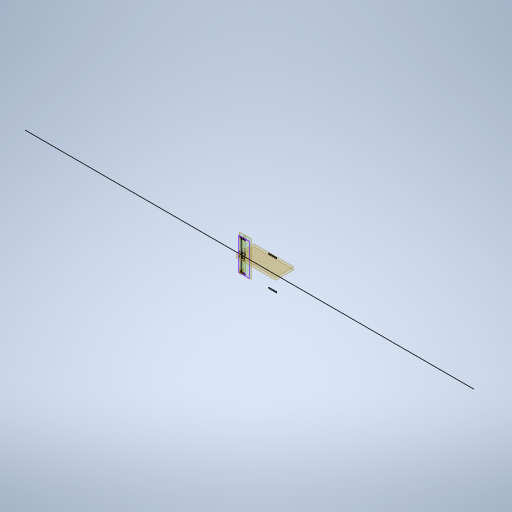
# Autodesk Inventor part: 4s
Saved by Autodesk Inventor 2024.2 (Build 282272000, 272)
## iProperties
Created: 2026-01-09
Part Number: 4s
Material: Типовые
Document SubType Name: Modeling
Designer: Service
Density: 1 g/cm^3
Appearance: По умолчанию
Author: Service
Autodesk Inventor part; units mm, degrees
ref_plane "YZ Plane" through (0, 0, 0) normal (1, 0, 0) x (0, 1, 0)
ref_plane "XZ Plane" through (0, 0, 0) normal (0, 1, 0) x (-1, 0, 0)
ref_plane "XY Plane" through (0, 0, 0) normal (0, 0, 1) x (1, 0, 0)
ref_plane "РабПлоскость1" through (0, 0, 0) normal (0, 0, 1) x (1, 0, 0)
sketch "Эскиз1" plane through (0, 0, 0) normal (0, 0, 1) x (1, 0, 0)
  line L0 (-20.21, 188.9707) -> (47.0583, 188.9707)
  line L1 (47.0583, 188.9707) -> (47.0583, -13.1291)
  line L2 (47.0583, -13.1291) -> (-20.21, -13.1291)
  line L3 (-20.21, -13.1291) -> (-20.21, 188.9707)
  line L4 (220, -6) -> (168.1947, -6)
  line L5 (168.1947, 0) -> (168.1947, -6)
  line L6 (168.1947, 0) -> (220, 0)
  line L7 (220, 0) -> (220, -6)
  line L8 (9.8053, -6) -> (-12, -6)
  line L9 (-12, -6) -> (-12, 0)
  line L10 (-12, 0) -> (9.8053, 0)
  line L11 (9.8053, 0) -> (9.8053, -6)
  line L12 (220, 180) -> (168.1947, 180)
  line L13 (168.1947, 186) -> (168.1947, 180)
  line L14 (168.1947, 186) -> (220, 186)
  line L15 (220, 186) -> (220, 180)
  line L16 (9.8053, 180) -> (-12, 180)
  line L17 (-12, 180) -> (-12, 186)
  line L18 (-12, 186) -> (9.8053, 186)
  line L19 (9.8053, 186) -> (9.8053, 180)
  line L20 (0, 180) -> (0, 0)
  line L21 (0, 0) -> (-6, 0)
  line L22 (-6, 0) -> (-6, 180)
  line L23 (-6, 180) -> (0, 180)
  circle A0 centre (-3, 175) radius 1.5
  circle A1 centre (-3, 5) radius 1.5
  line L24 (9.8053, -6) -> (24.8871, -6)
  line L25 (24.8871, -6) -> (24.8871, 0)
  line L26 (24.8871, 0) -> (9.8053, 0)
  line L27 (9.8053, 0) -> (9.8053, -6)
  line L28 (9.8053, 180) -> (24.8871, 180)
  line L29 (24.8871, 180) -> (24.8871, 188.9707)
  line L30 (24.8871, 188.9707) -> (9.8053, 188.9707)
  line L31 (9.8053, 188.9707) -> (9.8053, 180)
  circle A2 centre (6, 75) radius 1.5
  circle A3 centre (6, 105) radius 1.5
  line L32 (-1364.1034, 90) -> (1460.214, 90)
  line L33 (9.8053, 186) -> (24.8871, 186)
  dimension "d0" = 3
  dimension "d1" = 3
  dimension "d2" = 6
  dimension "d3" = 6
  dimension "d4" = 15
  dimension "d5" = 15
  constraints: 68 end point, 14 horizontal, 10 vertical, 6 parallel, 4 centre point, 4 perpendicular, 3 point on line, 25 other
  measures "d0" diameter of A3
  measures "d1" diameter of A2
  measures "d2" distance from line of L20 A2.centre
  measures "d3" distance from line of L20 A3.centre
  measures "d4" distance from line of L32 A2.centre
  measures "d5" distance from line of L32 A3.centre
ref_plane "РабПлоскость2" through (104, 75, -42) normal (0, 1, 0) x (-1, 0, 0)
sketch "Эскиз2" plane through (104, 75, -42) normal (0, 1, 0) x (-1, 0, 0)
  line L0 (104, 42) -> (104, 26.1085)
  line L1 (104, 26.1085) -> (90.5759, 39.2974)
  line L2 (90.5759, 39.2974) -> (104, 39.2974)
  constraints: 6 end point, 1 perpendicular, 1 point on line, 1 vertical
extrude "Выдавливание2" add sketch "Эскиз2" along normal mid plane 30
ref_plane "РабПлоскость3" through (104, 90, -42) normal (0, 1, 0) x (-1, 0, 0)
mirror "Зеркальное отражение1" about plane through (104, 90, -42) normal (0, 1, 0) of "Выдавливание2"
ref_plane "РабПлоскость7" through (0, 0, 0) normal (0, 0, 1) x (1, 0, 0)
sketch "Эскиз3" plane through (0, 0, 0) normal (0, 0, 1) x (1, 0, 0)
  line L0 (47.0583, 188.9707) -> (-20.21, 188.9707) projected
  line L1 (-20.21, 188.9707) -> (-20.21, -13.1291) projected
  line L2 (-20.21, -13.1291) -> (47.0583, -13.1291) projected
  line L3 (47.0583, -13.1291) -> (47.0583, 188.9707) projected
  circle A0 centre (6, 105) radius 1.5 projected
  circle A1 centre (6, 75) radius 1.5 projected
  line L4 (-12, 186) -> (24.8871, 186) projected
  line L5 (24.8871, 186) -> (24.8871, 180) projected
  line L6 (24.8871, 180) -> (0, 180) projected
  line L7 (0, 180) -> (0, 0) projected
  line L8 (0, 0) -> (24.8871, 0) projected
  line L9 (24.8871, 0) -> (24.8871, -6) projected
  line L10 (24.8871, -6) -> (-12, -6) projected
  line L11 (-12, -6) -> (-12, 0) projected
  line L12 (-12, 0) -> (-6, 0) projected
  line L13 (-6, 0) -> (-6, 180) projected
  line L14 (-6, 180) -> (-12, 180) projected
  line L15 (-12, 180) -> (-12, 186) projected
extrude "Выдавливание3" cut sketch "Эскиз3" against normal blind 13.891 contours A0 | A1
ref_plane "РабПлоскость4" through (0, 0, -10) normal (0, 0, -1) x (-1, 0, 0)
sketch "Эскиз4" plane through (0, 0, -10) normal (0, 0, -1) x (-1, 0, 0)
  line L0 (0, 60) -> (-13.4241, 60) projected
  line L1 (0, 120) -> (0, 60) projected
  line L2 (0, 120) -> (-13.4241, 120) projected
  circle A0 centre (-6, 105) radius 3.0499
  line L3 (-13.4241, 60) -> (-13.4241, 120) projected
  point P0 (0, 0)
  constraints: 1 centre point
extrude "Выдавливание4" cut sketch "Эскиз4" along normal blind 30 contours A0
mirror "Зеркальное отражение2" about plane through (104, 90, -42) normal (0, 1, 0) of "Выдавливание4"
ref_plane "РабПлоскость6" through (0, 0, 0) normal (-1, 0, 0) x (0, 0, 1)
sketch "Эскиз5" plane through (0, 0, 0) normal (-1, 0, 0) x (0, 0, 1)
  circle A0 centre (-10, 95) radius 1.3
  circle A1 centre (-10, 85) radius 1.3
  line L0 (-19.0698, 90) -> (3.1783, 90) projected
  line L1 (-3, -13.1291) -> (-3, 188.9707) projected
  point P0 (0, 0)
  dimension "d16" = 2.6
  dimension "d17" = 5
  dimension "d18" = 5
  dimension "d19" = 2.6
  dimension "d20" = 7
  dimension "d21" = 7
  constraints: 2 centre point
  measures "d16" diameter of A1
  measures "d17" distance from line of L0 A1.centre
  measures "d18" distance from line of L0 A0.centre
  measures "d19" diameter of A0
  measures "d20" distance from line of L1 A0.centre
  measures "d21" distance from line of L1 A1.centre
extrude "Выдавливание5" cut sketch "Эскиз5" against normal up to surface surface through (13.4241, 75, -2.7026) normal (0.7008276, 0, -0.7133306)
ref_plane "РабПлоскость5" through (4.6, 0, 0) normal (-1, 0, 0) x (0, 0, 1)
sketch "Эскиз6" plane through (4.6, 0, 0) normal (-1, 0, 0) x (0, 0, 1)
  circle A0 centre (-10, 85) radius 1.3 projected
  circle A1 centre (-10, 95) radius 1.3 projected
  line L0 (-3, 120) -> (-15.8915, 120) projected
  line L1 (-15.8915, 120) -> (-15.8915, 60) projected
  line L2 (-3, 60) -> (-15.8915, 60) projected
  line L3 (-3, 0) -> (-3, 60) projected
  line L4 (0, 0) -> (-3, 0) projected
  line L5 (0, 180) -> (0, 0) projected
  line L6 (0, 180) -> (-3, 180) projected
  line L7 (-3, 120) -> (-3, 180) projected
  circle A2 centre (-10, 85) radius 2.75
  circle A3 centre (-10, 95) radius 2.75
  point P0 (0, 0)
  dimension "d25" = 5.5
  dimension "d26" = 5.5
  constraints: 2 centre point, 2 coincident
  measures "d25" diameter of A2
  measures "d26" diameter of A3
extrude "Выдавливание6" cut sketch "Эскиз6" against normal blind 10 contours A0 | A2 | A3
